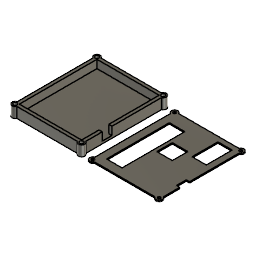
case (Autodesk Fusion 360 design; units mm, degrees)
part number: 2026-06-06-17-13-07-848
Autodesk Fusion 360 part; units mm, degrees
note: some values were not read from the file. Set by a fixed rule: which sketch regions a step uses.
sketch "Esboço1" plane through (0, 0, 0) normal (0, 0, 1) x (1, 0, 0)
  line L0 (0, 0) -> (76.2, 0)
  line L1 (76.2, 0) -> (76.2, -95.25)
  line L2 (76.2, -95.25) -> (0, -95.25)
  line L3 (0, -95.25) -> (0, 0)
  line L4 (4.895, -11.325) -> (23.945, -11.325)
  line L5 (23.945, -11.325) -> (23.945, -88.875)
  line L6 (23.945, -88.875) -> (4.895, -88.875)
  line L7 (4.895, -88.875) -> (4.895, -11.325)
  line L8 (28.114, -30.825) -> (47.164, -30.825)
  line L9 (47.164, -30.825) -> (47.164, -49.875)
  line L10 (47.164, -49.875) -> (28.114, -49.875)
  line L11 (28.114, -49.875) -> (28.114, -30.825)
  line L12 (72.965, -1.764) -> (55.465, -1.764)
  line L13 (55.465, -1.764) -> (55.465, -33.571)
  line L14 (55.465, -33.571) -> (72.965, -33.571)
  line L15 (72.965, -33.571) -> (72.965, -1.764)
  line L16 (76.6, 0.4) -> (76.6, -95.65)
  line L17 (76.6, -95.65) -> (-0.4, -95.65)
  line L18 (-0.4, -95.65) -> (-0.4, 0.4)
  line L19 (-0.4, 0.4) -> (76.6, 0.4)
  line L20 (80.6, 4.4) -> (80.6, -99.65)
  line L21 (80.6, -99.65) -> (-4.4, -99.65)
  line L22 (-4.4, -99.65) -> (-4.4, 4.4)
  line L23 (-4.4, 4.4) -> (80.6, 4.4)
  circle A0 centre (-2.8939, 2.9946) radius 2.35
  circle A1 centre (-2.8939, 2.9946) radius 4
  circle A2 centre (-3.158, -97.9444) radius 2.35
  circle A3 centre (-3.158, -97.9444) radius 4
  circle A4 centre (-2.8939, 2.9946) radius 2.35
  circle A5 centre (-2.8939, 2.9946) radius 4
  circle A6 centre (-2.8939, 2.9946) radius 2.35
  circle A7 centre (-2.8939, 2.9946) radius 4
  circle A8 centre (79, 3) radius 2.35
  circle A9 centre (79, 3) radius 4
  circle A10 centre (79, -98) radius 2.35
  circle A11 centre (79, -98) radius 4
  line L24 (69.403, -72.144) -> (69.403, -63.144)
  line L25 (80.6, -37.338) -> (76.2, -37.338)
  line L26 (80.6, -61.995) -> (76.6, -61.995)
  line L27 (80.6, -73.995) -> (76.6, -73.995)
  dimension "d1" = 76.2
  dimension "d2" = 95.25
  dimension "d5" = 19.05
  dimension "d6" = 77.55
  dimension "d9" = 19.05
  dimension "d13" = 17.5
  dimension "d14" = 31.807
  dimension "d15" = -0.4
  dimension "d16" = -4
  dimension "d18" = 4.7
  dimension "d19" = 8
  dimension "d20" = 4.7
  dimension "d21" = 8
  dimension "d22" = 4.7
  dimension "d23" = 8
  dimension "d24" = 4.7
  dimension "d25" = 8
  dimension "d28" = 4.7
  dimension "d29" = 8
  dimension "d30" = 4.7
  dimension "d31" = 8
  dimension "d34" = 9
  dimension "d35" = 12
  constraint horizontal L0
  constraint vertical L1
  constraint horizontal L2
  constraint vertical L3
  constraint coincident L0.start L3.end
  constraint horizontal L4
  constraint vertical L5
  constraint horizontal L6
  constraint vertical L7
  constraint horizontal L8
  constraint vertical L9
  constraint horizontal L10
  constraint vertical L11
  constraint horizontal L12
  constraint vertical L13
  constraint horizontal L14
  constraint vertical L15
  constraint concentric A0 A1
  constraint concentric A2 A3
  constraint concentric A4 A5
  constraint concentric A6 A7
  constraint concentric A8 A9
  constraint concentric A10 A11
  constraint coincident L20 L25.start
  constraint coincident L1 L25.end
  constraint perpendicular L1 L25
  constraint coincident L20 L26.start
  constraint coincident L16 L26.end
  constraint perpendicular L16 L26
  constraint coincident L20 L27.start
  constraint coincident L16 L27.end
  constraint perpendicular L16 L27
  measures "d1" distance of L0.start L0.end
  measures "d2" distance of L0.start L2.end
  measures "d5" distance of L4.start L4.end
  measures "d6" distance of L4.start L6.end
  measures "d9" distance of L8.start L8.end
  measures "d13" distance of L12.start L12.end
  measures "d14" distance of L12.start L14.end
  measures "d18" diameter of A0
  measures "d19" diameter of A1
  measures "d20" diameter of A2
  measures "d21" diameter of A3
  measures "d22" diameter of A4
  measures "d23" diameter of A5
  measures "d24" diameter of A6
  measures "d25" diameter of A7
  measures "d28" diameter of A8
  measures "d29" diameter of A9
  measures "d30" diameter of A10
  measures "d31" diameter of A11
  measures "d34" distance of L24.start L24.end
  measures "d35" distance of L26.start L27.start
extrude "Extrusão1" add sketch "Esboço1" along normal blind 3 contours L0 L1 L2 L3 L16 L17 L18 L19 A1 A3 A5 A7 A9 A11 L25 | L0 L1 L2 L3 A11 | L1 L16 A11 L25 | L1 L2 A11 | L1 L2 L16 L17 A11 | L16 L20 L25 L26 | L16 L20 A9 L25 | L17 L21 A3 A11 | L16 L17 L20 L21 A10 A11 | L16 L20 A11 L27 | L16 L19 A9 | L16 L19 L20 L23 A8 A9 | L17 L18 L21 L22 A2 A3 | L17 L18 A3 | L20 L21 A10 A11 | L19 L23 A1 A5 A7 A9 | L20 L23 A8 A9 | L18 L22 A1 A3 A5 A7 | L20 L21 A10 | L20 L21 A10 | L21 L22 A2 A3 | L18 L19 A1 A5 A7 | L18 L19 L22 L23 A0 A1 A4 A5 A6 A7 | L20 L23 A8 | L20 L23 A8 | L21 L22 A2 | L21 L22 A2 | L22 L23 A0 A1 A4 A5 A6 A7 | L22 L23 A0 A4 A6 | L22 L23 A0 A4 A6 | L4 L5 L6 L7 | L8 L9 L10 L11 | L12 L13 L14 L15 makes body 1
extrude "Extrusão2" add sketch "Esboço1" along normal blind 10 separate body contours L16 L20 L25 L26 | L16 L20 A9 L25 | L17 L21 A3 A11 | L16 L17 L20 L21 A10 A11 | L16 L20 A11 L27 | L16 L19 L20 L23 A8 A9 | L17 L18 L21 L22 A2 A3 | L20 L21 A10 A11 | L19 L23 A1 A5 A7 A9 | L20 L23 A8 A9 | L18 L22 A1 A3 A5 A7 | L21 L22 A2 A3 | L18 L19 L22 L23 A0 A1 A4 A5 A6 A7 | L22 L23 A0 A1 A4 A5 A6 A7 makes body 2
extrude "Extrusão3" add sketch "Esboço1" along normal blind 3 separate body contours L16 L20 L26 L27 makes body 3
sketch "Esboço2" plane through (0, 0, 0) normal (0, 0, 1) x (1, 0, 0)
  line L0 (75.3562, -99.65) -> (0.4602, -99.65)
  arc A0 (-4.4, -94.1421) -> (0.4602, -99.65) centre (-3.158, -97.9444) ccw
  line L1 (-4.4, -94.1421) -> (-4.4, -0.711)
  arc A1 (0.8511, 4.4) -> (-4.4, -0.711) centre (-2.8939, 2.9946) ccw
  line L2 (0.8511, 4.4) -> (75.253, 4.4)
  arc A2 (80.6, -0.6661) -> (75.253, 4.4) centre (79, 3) ccw
  line L3 (80.6, -0.6661) -> (80.6, -61.995)
  line L4 (80.6, -61.995) -> (76.6, -61.995)
  line L5 (76.6, -61.995) -> (76.6, -73.995)
  line L6 (80.6, -73.995) -> (76.6, -73.995)
  line L7 (80.6, -73.995) -> (80.6, -94.3339)
  arc A3 (75.3562, -99.65) -> (80.6, -94.3339) centre (79, -98) ccw
  line L8 (80.6, -61.995) -> (80.6, -73.995)
  line L9 (80.6, -73.995) -> (76.6, -73.995)
  line L10 (76.6, -61.995) -> (76.6, -73.995)
  line L11 (80.6, -61.995) -> (76.6, -61.995)
  circle A4 centre (-2.8939, 2.9946) radius 1.75
  circle A5 centre (79, 3) radius 1.75
  circle A6 centre (-3.158, -97.9444) radius 1.75
  circle A7 centre (79, -98) radius 1.75
  line L12 (4.895, -11.325) -> (23.945, -11.325)
  line L13 (23.945, -11.325) -> (23.945, -88.875)
  line L14 (23.945, -88.875) -> (4.895, -88.875)
  line L15 (4.895, -88.875) -> (4.895, -11.325)
  line L16 (28.114, -30.825) -> (47.164, -30.825)
  line L17 (47.164, -30.825) -> (47.164, -49.875)
  line L18 (47.164, -49.875) -> (28.114, -49.875)
  line L19 (28.114, -49.875) -> (28.114, -30.825)
  line L20 (76.2, 0) -> (72.965, 0)
  line L21 (76.2, -1.764) -> (76.2, 0)
  line L22 (72.965, -1.764) -> (55.465, -1.764)
  line L23 (55.465, -1.764) -> (55.465, -33.571)
  line L24 (55.465, -33.571) -> (72.965, -33.571)
  line L25 (72.965, -33.571) -> (72.965, -1.764)
  dimension "d42" = 3.5
  dimension "d43" = 3.5
  dimension "d44" = 3.5
  dimension "d45" = 3.5
  dimension "d48" = 19.05
  dimension "d49" = 19.05
  dimension "d50" = 3.235
  dimension "d51" = 1.764
  dimension "d52" = 17.5
  dimension "d53" = 31.807
  constraint concentric A1 A4
  constraint coincident A2.centre A5.centre
  constraint coincident A0.centre A6.centre
  constraint concentric A3 A7
  constraint horizontal L12
  constraint vertical L13
  constraint horizontal L14
  constraint vertical L15
  constraint horizontal L16
  constraint vertical L17
  constraint horizontal L18
  constraint vertical L19
  constraint horizontal L20
  constraint horizontal L22
  constraint vertical L23
  constraint horizontal L24
  constraint vertical L25
  measures "d42" diameter of A4
  measures "d43" diameter of A5
  measures "d44" diameter of A6
  measures "d45" diameter of A7
  measures "d48" distance of L16.start L16.end
  measures "d49" distance of L16.start L18.end
  measures "d50" distance of L20.start L20.end
  measures "d51" distance of L20.start L21.start
  measures "d52" distance of L22.start L22.end
  measures "d53" distance of L22.start L24.end
extrude "Extrusão4" add sketch "Esboço2" against normal blind 1.5 separate body contours L0 A0 L1 A1 L2 A2 L3 L4 L5 L6 L7 A3 L9 L10 L11 makes body 4
move_body "Mover1" bodies 4 to x (1, 0, 0) y (0, 1, 0) z (0, 0, 1) at (0, 0, 21)
extrude "Extrusão5" add 1 faces at (80.6, -65.995, 2) along direction (-1, 0, 0) blind 4 on bodies 3 bodies 1 3
move_body "Mover2" bodies 2 to x (1, 0, 0) y (0, 1, 0) z (0, 0, 1) at (0, 0, 4)
move_body "Mover3" bodies 2 to x (1, 0, 0) y (0, 1, 0) z (0, 0, 1) at (0, 0, -1)
extrude "Extrusão6" add 2 faces at (80.6, -31.8887, 1) (80.6, -12.89, 6.3333) along direction (-1, 0, 0) blind 4 on bodies 1 2 bodies 1 2
move_face "MoverFace1" by (0, 40, 0) 1 faces at (49.2363, -70.915, 21) on bodies 4
move_face "MoverFace2" by (0, 160, 0) 1 faces at (49.2363, -70.915, 21) on bodies 4
move_body "Mover4" bodies 4 to x (1, 0, 0) y (0, 1, 0) z (0, 0, 1) at (0, 0, -7)
move_body "Mover5" bodies 4 to x (1, 0, 0) y (0, 1, 0) z (0, 0, 1) at (0, 0, 0.5)
move_body "Mover6" bodies 4 to x (1, 0, 0) y (0, 1, 0) z (0, 0, 1) at (96, 0, -13)
named bodies: "caixa bottom", "tampa top"
